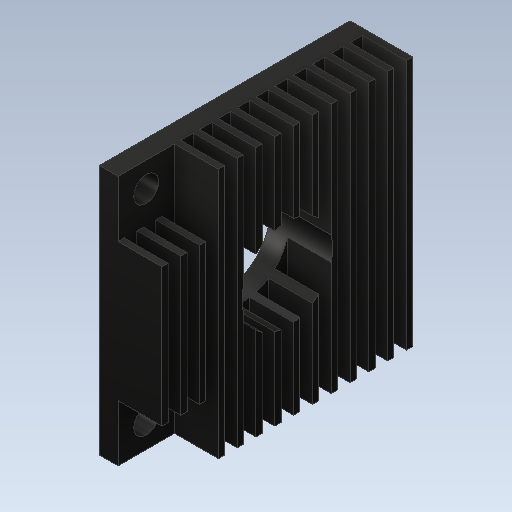
# Autodesk Inventor part: 36_radiator
Saved by Autodesk Inventor 2020.2 (Build 242310000, 310)
## iProperties
Created: 2017-11-11
Part Number: 36_radiator
Material: Ogólny
Document SubType Name: Modeling
Designer: Haras
Density: 1 g/cm^3
Appearance: Domyślna
Author: Haras
Autodesk Inventor part; units mm, degrees
ref_plane "YZ Plane" through (0, 0, 0) normal (1, 0, 0) x (0, 1, 0)
ref_plane "XZ Plane" through (0, 0, 0) normal (0, 1, 0) x (-1, 0, 0)
ref_plane "XY Plane" through (0, 0, 0) normal (0, 0, 1) x (1, 0, 0)
sketch "Szkic1" plane through (0, 0, 0) normal (1, 0, 0) x (0, 1, 0)
  line L0 (20, 20) -> (-20, 20)
  line L1 (-20, 20) -> (-20, -20)
  line L2 (-20, -20) -> (20, -20)
  line L3 (20, -20) -> (20, 20)
  line L4 (20, 0) -> (0, 0) construction
  line L5 (0, 0) -> (0, -20) construction
  dimension "d0" = 40
  dimension "d1" = 40
  constraints: 12 end point, 2 horizontal, 2 midpoint, 2 parallel, 1 perpendicular, 1 vertical
  measures "d0" distance of L2.end L0.start
  measures "d1" distance of L1.end L2.end
extrude "Wyciągnięcie proste1" add sketch "Szkic1" along normal blind 2
sketch "Szkic4" plane through (0, 20, 20) normal (0, 1, 0) x (1, 0, 0)
  line L0 (0, 40) -> (2, 40) projected
  line L1 (2, 40) -> (10, 40)
  line L2 (10, 40) -> (10, 39)
  line L3 (10, 39) -> (3, 39)
  line L4 (3, 39) -> (3, 37)
  line L5 (3, 37) -> (2, 37)
  line L6 (2, 40) -> (2, 37)
  line L7 (2, 0) -> (2, 40) projected
  point P0 (0, 20)
  dimension "d27" = 8
  dimension "d29" = 2
  dimension "d30" = 1
  dimension "d31" = 1
  constraints: 12 end point, 4 perpendicular, 1 collinear, 1 horizontal
  measures "d27" distance of L0.end L1.end
  measures "d29" distance of L3.end L4.end
  measures "d30" distance of L1.end L2.end
  measures "d31" distance of L4.end L5.end
extrude "Wyciągnięcie proste2" add sketch "Szkic4" against normal up to surface (40 mm away)
pattern_linear "Szyk prostokątny1" count 13 spacing 3 along (0, 0, 1) of "Wyciągnięcie proste2"
sketch "Szkic5" plane through (0, 20, 20) normal (0, 1, 0) x (1, 0, 0)
  line L0 (2, 1) -> (2, 0) projected
  line L1 (2, 1) -> (10, 1)
  line L2 (10, 1) -> (10, 0)
  line L3 (10, 0) -> (2, 0)
  line L4 (2, 0) -> (2, 1)
  line L5 (10, 3) -> (10, 4) projected
  line L6 (0, 0) -> (2, 0) projected
  point P0 (0, 20)
  point P1 (1, 0)
  constraints: 8 end point, 2 parallel, 1 collinear, 1 horizontal, 1 horizontal alignment, 1 midpoint, 1 perpendicular
extrude "Wyciągnięcie proste3" add sketch "Szkic5" against normal up to surface (40 mm away)
sketch "Szkic6" plane through (0, 0, 0) normal (-1, 0, 0) x (0, 0, 1)
  point P0 (0, 0)
  point P1 (0, 0)
  constraints: 1 coincident
hole "Otwór1" at (0, 0, 0) direction (1, 0, 0) diameter 14.5 end through all
sketch "Szkic7" plane through (0, 0, 0) normal (-1, 0, 0) x (0, 0, 1)
  line L0 (0, 0) -> (-20, 0) construction
  line L1 (-20, -20) -> (-20, 20) projected
  line L2 (20, 20) -> (20, -20) projected
  point P0 (15.5, -16)
  point P1 (15.5, 16)
  dimension "d46" = 32
  dimension "d47" = 4.5
  constraints: 2 end point, 1 midpoint, 1 symmetric about line, 1 vertical alignment
  measures "d46" distance of point (15.5, 16) point (15.5, -16)
  measures "d47" distance from line of L2 point (15.5, -16)
hole "Otwór2" at (0, -16, 15.5) at (0, 16, 15.5) direction (1, 0, 0) diameter 4 end through all
sketch "Szkic8" plane through (10, 20, 20) normal (1, 0, 0) x (0, 0, -1)
  line L0 (0, 0) -> (0, -40) projected
  line L1 (7, 0) -> (0, 0)
  line L2 (0, 0) -> (0, -9)
  line L3 (0, -9) -> (7, -9)
  line L4 (7, -9) -> (7, 0)
  line L5 (7, 0) -> (7, -40) projected
  line L6 (0, -40) -> (7, -40)
  line L7 (7, -40) -> (7, -31)
  line L8 (7, -31) -> (0, -31)
  line L9 (0, -31) -> (0, -40)
  point P0 (20, -20)
  dimension "d56" = 9
  dimension "d57" = 9
  constraints: 16 end point, 4 parallel, 3 point on line, 2 horizontal, 2 perpendicular, 1 collinear
  measures "d56" distance between parallel lines of L1 L3
  measures "d57" distance between parallel lines of L6 L8
extrude "Wyciągnięcie proste4" cut sketch "Szkic8" against normal up to surface (7 mm away) contours L1 L4 L3 L0 | L8 L5 L6 L0
